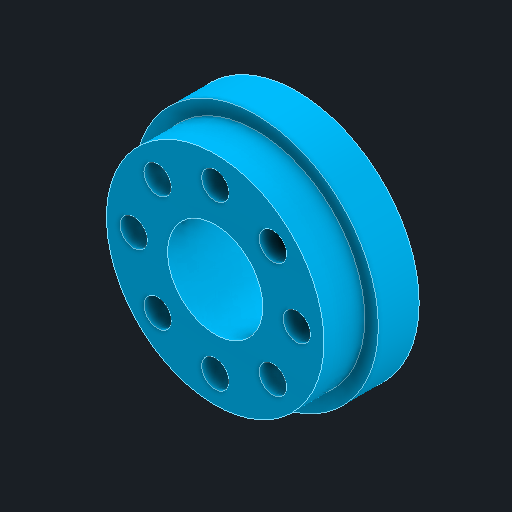
# Autodesk Inventor part: SecondStageArmClamp
Saved by Autodesk Inventor 2025 (Build 290162000, 162)
## iProperties
Created: 2024-01-28
Part Number: SecondStageArmClamp
Material: PC/ABS Plastic
Document SubType Name: Modeling
Designer: avsar
Density: 1.1 g/cm^3
Appearance: Sky Blue Medium
Author: avsar
Autodesk Inventor part; units mm, degrees
ref_plane "YZ Plane" through (0, 0, 0) normal (1, 0, 0) x (0, 1, 0)
ref_plane "XZ Plane" through (0, 0, 0) normal (0, 1, 0) x (-1, 0, 0)
ref_plane "XY Plane" through (0, 0, 0) normal (0, 0, 1) x (1, 0, 0)
sketch "Sketch1" plane through (0, 0, 0) normal (0, 0, 1) x (1, 0, 0)
  circle A0 centre (0, 0) radius 18
  dimension "d0" = 36
  constraints: 1 centre point, 1 coincident
  measures "d0" diameter of A0
extrude "Extrusion1" add sketch "Sketch1" along normal blind 6
sketch "Sketch2" plane through (0, 0, 6) normal (0, 0, 1) x (1, 0, 0)
  circle A0 centre (0, 0) radius 16
  dimension "d3" = 32
  constraints: 1 centre point, 1 coincident
  measures "d3" diameter of A0
extrude "Extrusion2" add sketch "Sketch2" along normal blind 6
sketch "Sketch3" plane through (0, 0, 12) normal (0, 0, 1) x (1, 0, 0)
  circle A0 centre (0, 0) radius 7
  circle A1 centre (-8.4853, 8.4853) radius 2
  circle A2 centre (-12, 0) radius 2
  circle A3 centre (-8.4853, -8.4853) radius 2
  circle A4 centre (0, -12) radius 2
  line L0 (-8.4853, 8.4853) -> (0, 0) construction
  line L1 (-7, 0) -> (0, 0) construction
  circle A5 centre (8.4853, -8.4853) radius 2
  circle A6 centre (12, 0) radius 2
  circle A7 centre (8.4853, 8.4853) radius 2
  circle A8 centre (0, 12) radius 2
  dimension "d6" = 14
  dimension "d7" = 4
  dimension "d12" = 360
  dimension "d16" = 45
  dimension "d17" = 12
  constraints: 8 centre point, 4 end point, 1 coincident, 1 horizontal, 1 horizontal alignment, 19 other
  measures "d7" diameter of A1
  measures "d16" angle of L0 L1
  measures "d17" distance of L0.start L0.end
extrude "Extrusion3" cut sketch "Sketch3" against normal through all
body "Solid1"
